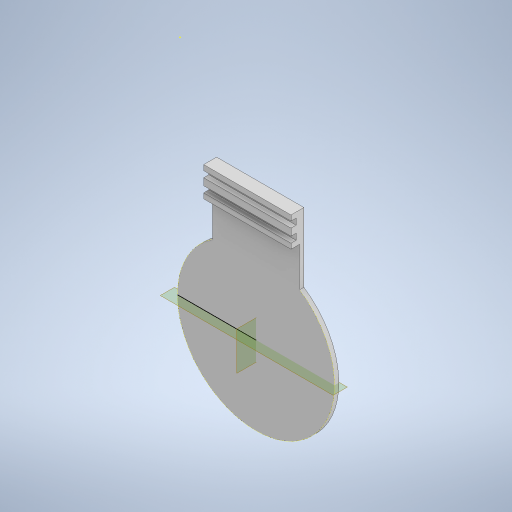
# Autodesk Inventor part: AnemoHolder
Saved by Autodesk Inventor 2023 (Build 270158000, 158)
## iProperties
Created: 2023-03-27
Part Number: AnemoHolder
Material: Générique
Document SubType Name: Modeling
Designer: eleves
Density: 1 g/cm^3
Appearance: Par défaut
Author: eleves
## iProperties of the stored document rainHolder_Impression 3D.ipt
Created: 2023-03-27
Part Number: rainHolder_Impression 3D
Material: Générique
Document SubType Name: Modeling
Designer: eleves
Density: 1 g/cm^3
Appearance: Par défaut
Author: eleves
Autodesk Inventor part; units mm, degrees
ref_plane "YZ Plane" through (0, 0, 0) normal (1, 0, 0) x (0, 1, 0)
ref_plane "XZ Plane" through (0, 0, 0) normal (0, 1, 0) x (-1, 0, 0)
ref_plane "XY Plane" through (0, 0, 0) normal (0, 0, 1) x (1, 0, 0)
sketch "Esquisse1" plane through (0, 0, 0) normal (0, 0, 1) x (1, 0, 0)
  line L0 (-65.5174, -57.3571) -> (-65.5174, -54.3571) construction
  line L1 (-65.5174, -57.3571) -> (68.5174, -57.3571) construction
  line L2 (68.5174, -54.3571) -> (68.5174, -57.3571) construction
  line L3 (68.5174, -54.3571) -> (-65.5174, -54.3571) construction
  line L4 (-65.5174, -65.3571) -> (-65.5174, -62.3571) construction
  line L5 (-65.5174, -65.3571) -> (68.5174, -65.3571) construction
  line L6 (68.5174, -62.3571) -> (68.5174, -65.3571) construction
  line L7 (68.5174, -62.3571) -> (-65.5174, -62.3571) construction
  line L8 (68.5174, -54.3571) -> (-65.5174, -65.3571) construction
  line L9 (-65.5174, -54.3571) -> (68.5174, -65.3571) construction
  line L10 (-65.5174, -61.8571) -> (68.5174, -61.8571)
  line L11 (68.5174, -61.8571) -> (68.5174, -57.8571)
  line L12 (68.5174, -57.8571) -> (-65.5174, -57.8571)
  line L13 (-65.5174, -57.8571) -> (-65.5174, -61.8571)
  line L14 (-65.5174, -61.8571) -> (68.5174, -57.8571) construction
  line L15 (68.5174, -61.8571) -> (-65.5174, -57.8571) construction
  line L16 (68.5174, -54.3571) -> (18.5174, -54.3571)
  line L17 (18.5174, -54.3571) -> (18.5174, -51.3571)
  line L18 (18.5174, -51.3571) -> (68.5174, -51.3571)
  line L19 (68.5174, -51.3571) -> (68.5174, -54.3571)
  line L20 (68.5174, -65.3571) -> (18.5174, -65.3571)
  line L21 (18.5174, -65.3571) -> (18.5174, -68.3571)
  line L22 (18.5174, -68.3571) -> (68.5174, -68.3571)
  line L23 (68.5174, -68.3571) -> (68.5174, -65.3571)
  line L24 (18.5174, -57.8571) -> (18.5174, -61.8571)
  point P0 (0, 0)
  point P1 (1.5, -59.8571)
  dimension "d1" = 0.5
  dimension "d2" = 50
  dimension "d3" = 3
  dimension "d4" = 3
  constraints: 34 end point, 6 parallel, 4 perpendicular, 3 horizontal, 3 midpoint, 3 point on line
  measures "d1" distance between parallel lines of L1 L12
  measures "d2" distance of L17.end L18.end
  measures "d3" distance of L18.end L2.start
  measures "d4" distance of L22.end L5.end
extrude "Extrusion1" add sketch "Esquisse1" along normal blind 2.9 contours L24 L12 L11 L10 | L16 L17 L18 L19 | L23 L22 L21 L20
sketch "Esquisse13" plane through (0, 0, 0) normal (0, 0, -1) x (-1, 0, 0)
  line L0 (-68.5174, -68.3571) -> (-68.5174, -65.3571) projected
  line L1 (-18.5174, -51.3571) -> (-68.5174, -51.3571)
  line L2 (-68.5174, -51.3571) -> (-68.5174, -68.3571)
  line L3 (-68.5174, -68.3571) -> (-18.5174, -68.3571)
  line L4 (-18.5174, -68.3571) -> (-18.5174, -51.3571)
  point P0 (0, 0)
  constraints: 8 end point, 2 parallel, 1 horizontal, 1 perpendicular
extrude "Extrusion12" add sketch "Esquisse13" along normal blind 2
sketch "Esquisse24" plane through (0, 0, -2) normal (0, 0, -1) x (-1, 0, 0)
  line L0 (-18.5174, -65.3571) -> (-18.5174, -68.3571) projected
  line L1 (-18.5174, -51.3571) -> (-68.5174, -51.3571) projected
  line L2 (-18.5174, -68.3571) -> (-68.5174, -68.3571)
  line L3 (-68.5174, -68.3571) -> (-68.5174, -51.3571)
  line L4 (-68.5174, -51.3571) -> (-18.5174, -51.3571)
  line L5 (-18.5174, -51.3571) -> (-18.5174, -68.3571)
  point P0 (0, 0)
  constraints: 8 end point, 2 parallel, 1 horizontal, 1 perpendicular
extrude "Extrusion21" add sketch "Esquisse24" along normal blind 5
sketch "Esquisse25" plane through (18.5174, -68.3571, 2.9) normal (0, -1, 0) x (1, 0, 0)
  line L0 (50, -9.9) -> (50, 0) projected
  line L1 (50, -9.9) -> (0, -9.9)
  line L2 (0, -9.9) -> (0, -4.95)
  line L3 (0, -4.95) -> (50, -4.95)
  line L4 (50, -4.95) -> (50, -9.9)
  line L5 (0, -9.9) -> (0, 0) construction
  point P0 (-18.5174, -2.9)
  constraints: 8 end point, 2 parallel, 1 collinear, 1 horizontal, 1 perpendicular
extrude "Extrusion22" add sketch "Esquisse25" along normal blind 15
sketch "Esquisse26" plane through (18.5174, -68.3571, -2.05) normal (0, 0, 1) x (1, 0, 0)
  line L0 (50, -15) -> (0, -15) projected
  line L1 (0, 0) -> (50, 0) projected
  line L2 (0, -15) -> (50, 0)
  line L3 (0, 0) -> (50, -15)
  line L4 (25, -7.5) -> (25, -60)
  circle A0 centre (25, -60) radius 45
  line L5 (0, -15) -> (50, -15) projected
  line L6 (0, -15) -> (0, -22.5834)
  line L7 (50, 0) -> (50, -15) projected
  line L8 (50, -15) -> (50, -22.5834)
  line L9 (0, -15) -> (25, -15)
  line L10 (25, -15) -> (50, -15)
  point P0 (-18.5174, 68.3571)
  dimension "d89" = 90
  constraints: 14 end point, 3 point on circle, 2 collinear, 2 midpoint, 2 tangent, 1 centre point, 1 coincident, 1 perpendicular, 1 vertical
  measures "d89" diameter of A0
extrude "Extrusion23" add sketch "Esquisse26" against normal up to surface (4.95 mm away) contours L8 A0 L0 | A0 L6 L0 | A0
sketch "Esquisse27" plane through (0, 0, -7) normal (0, 0, -1) x (-1, 0, 0)
  line L0 (-18.5174, -51.3571) -> (-18.5174, -90.9406) projected
  line L1 (-18.5174, -51.3571) -> (-68.5174, -51.3571) projected
  line L2 (-68.5174, -51.3571) -> (-68.5174, -90.9406) projected
  arc A0 (-68.5174, -90.9406) -> (-18.5174, -90.9406) centre (-43.5174, -128.3571) ccw projected
  point P0 (0, 0)
extrude "Extrusion24" cut sketch "Esquisse27" against normal blind 2.5
sketch "Esquisse28" plane through (18.5174, -68.3571, -2.05) normal (0, 0, 1) x (1, 0, 0)
  arc A0 (0, -22.5834) -> (50, -22.5834) centre (25, -60) ccw construction
  line L0 (25, -60) -> (-20, -60)
  point P0 (-18.5174, 68.3571)
  constraints: 2 end point, 1 horizontal, 1 point on circle
ref_plane "Plan de construction5" through (43.5174, -128.3571, -2.05) normal (0, -1, 0) x (1, 0, 0)
ref_plane "Plan de construction6" through (43.5174, -128.3571, -2.05) normal (-1, 0, 0) x (0, -1, 0)
